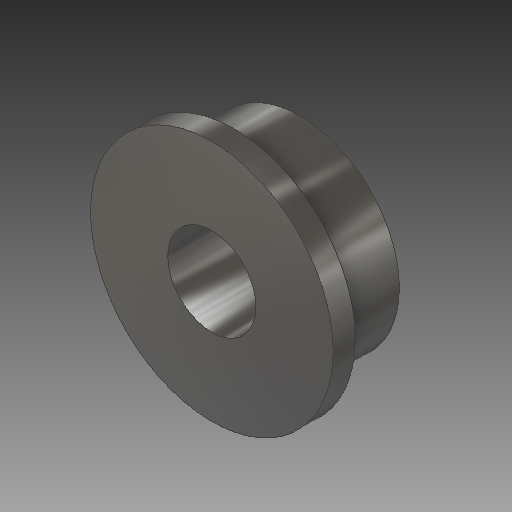
# Autodesk Inventor part: ベアリングフランジ付き040904
Saved by Autodesk Inventor 2020 (Build 240168000, 168)
## iProperties
Created: 2018-09-17
Part Number: ベアリングフランジ付き040904
Material: 鋼、高強度、低合金
Document SubType Name: Modeling
Designer: 雪村
Density: 7.85 g/cm^3
Appearance: 鋼 - つや出し
Mass: 1.84961 g
Surface Area: 3.3458 cm^2
Volume: 0.235619 cm^3
Author: 雪村
Autodesk Inventor part; units mm, degrees
ref_plane "YZ Plane" through (0, 0, 0) normal (1, 0, 0) x (0, 1, 0)
ref_plane "XZ Plane" through (0, 0, 0) normal (0, 1, 0) x (-1, 0, 0)
ref_plane "XY Plane" through (0, 0, 0) normal (0, 0, 1) x (1, 0, 0)
sketch "スケッチ1" plane through (0, 0, 0) normal (0, 0, 1) x (1, 0, 0)
  circle A0 centre (0, 0) radius 2
  circle A1 centre (0, 0) radius 4.5
  dimension "d0" = 4
  dimension "d1" = 9
  constraints: 2 centre point, 2 coincident
  measures "d0" diameter of A0
  measures "d1" diameter of A1
extrude "押し出し1" add sketch "スケッチ1" along normal blind 4
sketch "スケッチ2" plane through (0, 0, 4) normal (0, 0, 1) x (1, 0, 0)
  circle A0 centre (0, 0) radius 2 projected
  circle A1 centre (0, 0) radius 5.5
  circle A2 centre (0, 0) radius 4.5 projected
  dimension "d7" = 1
  constraints: 1 centre point, 1 coincident
  measures "d7" radial gap between concentric circles of A2 A1
extrude "押し出し2" add sketch "スケッチ2" against normal blind 1 contours A1 | A2
